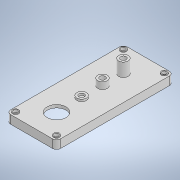
# Autodesk Inventor part: Основание сервы
Saved by Autodesk Inventor 2020 (Build 240168000, 168)
## iProperties
Created: 2021-09-05
Part Number: Основание сервы
Material: Типовые
Document SubType Name: Modeling
Designer: Антон
Density: 1 g/cm^3
Appearance: По умолчанию
Author: Антон
Autodesk Inventor part; units mm, degrees
ref_plane "YZ Plane" through (0, 0, 0) normal (1, 0, 0) x (0, 1, 0)
ref_plane "XZ Plane" through (0, 0, 0) normal (0, 1, 0) x (-1, 0, 0)
ref_plane "XY Plane" through (0, 0, 0) normal (0, 0, 1) x (1, 0, 0)
sketch "Эскиз1" plane through (0, 0, 0) normal (0, 1, 0) x (-1, 0, 0)
  line L0 (0, 0) -> (12, 0)
  line L1 (12, 0) -> (12, -28)
  line L2 (12, -28) -> (0, -28)
  line L3 (0, -28) -> (0, 0)
  circle A0 centre (6, -12) radius 0.65
  circle A1 centre (6, -17) radius 0.65
  circle A2 centre (6, -22) radius 0.65
  line L4 (6, -12) -> (6, -17) construction
  line L5 (6, -17) -> (6, -22) construction
  line L6 (6, -6) -> (6, 0) construction
  line L7 (6, -12) -> (12, -12) construction
  circle A3 centre (6, -17) radius 1.15
  circle A4 centre (6, -12) radius 1.15
  circle A5 centre (6, -22) radius 1.15
  circle A6 centre (6, -6) radius 2.25
  line L8 (6, -12) -> (6, -6) construction
  line L9 (6, -22) -> (6, -28) construction
  point P0 (12, -14)
  dimension "d1" = 5
  dimension "d4" = 6
  dimension "d5" = 1.3
  dimension "d6" = 0.5
  dimension "d30" = 6
  dimension "d31" = 4.5
  constraints: 20 end point, 7 centre point, 4 equal radius, 3 coincident, 3 equal length, 3 midpoint, 2 collinear, 2 parallel, 2 perpendicular, 2 point on line, 2 vertical, 1 concentric, 1 horizontal, 1 vertical alignment
  measures "d1" distance of L4.start L4.end
  measures "d4" distance of L4.start L7.end
  measures "d5" diameter of A1
  measures "d6" radial gap between concentric circles of A3 A1
  measures "d30" distance of L8.start L6.start
  measures "d31" diameter of A6
extrude "Выдавливание1" add sketch "Эскиз1" against normal blind 2 contours L0 L1 L2 L3 | A0 | A1 | A2 | A3 | A4 | A5 | A6
extrude "Выдавливание2" add sketch "Эскиз1" along normal blind 0.5 contours A4
extrude "Выдавливание4" add sketch "Эскиз1" along normal blind 1.6 contours A3
extrude "Выдавливание5" add sketch "Эскиз1" along normal blind 3.2 contours A5
sketch "Эскиз2" plane through (-6, 1.6, -17) normal (0, 1, 0) x (1, 0, 0)
  circle A0 centre (0, 0) radius 0.65 projected
  point P0 (6, -17)
extrude "Выдавливание3" cut sketch "Эскиз2" against normal through all
extrude "Выдавливание7" cut sketch "Эскиз1" against normal through all contours A6
sketch "Эскиз7" plane through (0, -2, 0) normal (0, -1, 0) x (1, 0, 0)
  circle A0 centre (-6, -6) radius 2.25 projected
  line L0 (-1, -10) -> (-11, -10)
  line L1 (-11, -10) -> (-11, -2)
  line L2 (-11, -2) -> (-1, -2)
  line L3 (-1, -2) -> (-1, -10)
  line L4 (-1, -10) -> (-11, -2) construction
  line L5 (-11, -10) -> (-1, -2) construction
  point P0 (0, 0)
  dimension "d34" = 10
  dimension "d35" = 8
  constraints: 12 end point, 2 midpoint, 2 parallel, 1 horizontal, 1 perpendicular
  measures "d34" distance of L1.end L2.end
  measures "d35" distance of L0.end L1.end
extrude "Выдавливание8" cut sketch "Эскиз7" against normal blind 1.3
sketch "Эскиз5" plane through (0, 0, 0) normal (0, 1, 0) x (1, 0, 0)
  circle A0 centre (-1.1, 1.1) radius 0.7
  line L0 (0, 0) -> (0, 28) projected
  line L1 (0, 0) -> (-12, 0) construction
  line L2 (-6, 0) -> (-6, 28) construction
  line L3 (-12, 28) -> (0, 28) construction
  line L4 (-12, 0) -> (-12, 28) construction
  line L5 (-12, 14) -> (0, 14) construction
  circle A1 centre (-10.9, 1.1) radius 0.7
  circle A2 centre (-1.1, 26.9) radius 0.7
  circle A3 centre (-10.9, 26.9) radius 0.7
  dimension "d17" = 1.1
  dimension "d18" = 1.4
  dimension "d19" = 1.1
  constraints: 4 centre point, 4 end point, 4 midpoint, 3 symmetric about line, 3 other
  measures "d17" distance from line of L0 A0.centre
  measures "d18" diameter of A0
  measures "d19" distance from line of L1 A0.centre
extrude "Выдавливание6" add sketch "Эскиз5" along normal blind 0.2
sketch "Эскиз6" plane through (-10.9, 0.2, -1.1) normal (0, 1, 0) x (1, 0, 0)
  circle A0 centre (0, 0) radius 0.7 projected
  circle A1 centre (9.8, 0) radius 0.7 projected
  circle A2 centre (9.8, 25.8) radius 0.7 projected
  circle A3 centre (0, 25.8) radius 0.7 projected
  point P0 (10.9, -1.1)
hole "Отверстие1" at (-10.9, 0.2, -1.1) at (-1.1, 0.2, -1.1) at (-10.9, 0.2, -26.9) at (-1.1, 0.2, -26.9) direction (0, -1, 0) diameter 1 end through all
fillet "Сопряжение1" radius 1 4 edges at (0, -1, 0) (-12, -1, 0) (0, -1, -28) (-12, -1, -28)
equation "\"d19\" = d17"
